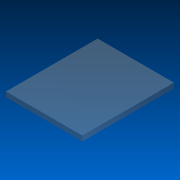
# Autodesk Inventor part: GoPro Hero 3 Screen
Saved by Autodesk Inventor 2015 (Build 190159000, 159)
## iProperties
Created: 2013-02-14
Material: Glass, Frosted
Document SubType Name: Modeling
Designer: sdarley
Density: 1 g/cm^3
Project: GoPro Hero 3 HD Camera
Description: GoPro Hero 3 Screen
Appearance: Satin
Author: sdarley
Title: GoPro Hero 3 Screen
Revision Number: 1
Autodesk Inventor part; units mm, degrees
ref_plane "YZ Plane" through (0, 0, 0) normal (1, 0, 0) x (0, 1, 0)
ref_plane "XZ Plane" through (0, 0, 0) normal (0, 1, 0) x (-1, 0, 0)
ref_plane "XY Plane" through (0, 0, 0) normal (0, 0, 1) x (1, 0, 0)
sketch "Sketch1" plane through (0, 0, 0) normal (0, 0, 1) x (1, 0, 0)
  line L0 (-7.5, -9) -> (7.5, -9)
  line L1 (7.5, -9) -> (7.5, 9)
  line L2 (7.5, 9) -> (-7.5, 9)
  line L3 (-7.5, 9) -> (-7.5, -9)
  line L4 (-7.5, -9) -> (7.5, 9) construction
  line L5 (7.5, -9) -> (-7.5, 9) construction
  point P0 (0, 0)
  dimension "d0" = 15
  dimension "d1" = 18
  constraints: 12 end point, 2 midpoint, 2 parallel, 1 horizontal, 1 perpendicular
  measures "d0" distance of L2.end L1.end
  measures "d1" distance of L1.end L0.end
extrude "Extrusion1" add sketch "Sketch1" along normal blind 1
body "Solid1"
